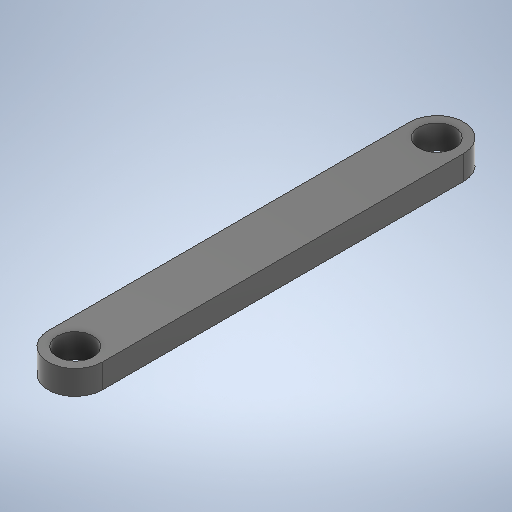
# Autodesk Inventor part: Servo connector
Saved by Autodesk Inventor 2025.2 (Build 292293000, 293)
## iProperties
Created: 2025-01-30
Part Number: Servo connector
Material: Generic
Document SubType Name: Modeling
Designer: caomi
Density: 1 g/cm^3
Appearance: Default
Author: caomi
Autodesk Inventor part; units mm, degrees
ref_plane "YZ Plane" through (0, 0, 0) normal (1, 0, 0) x (0, 1, 0)
ref_plane "XZ Plane" through (0, 0, 0) normal (0, 1, 0) x (-1, 0, 0)
ref_plane "XY Plane" through (0, 0, 0) normal (0, 0, 1) x (1, 0, 0)
sketch "Sketch1" plane through (0, 0, 0) normal (0, 1, 0) x (-1, 0, 0)
  line L0 (0, 15) -> (0, -15) construction
  line L1 (-2.25, 15) -> (-2.25, -15)
  line L2 (2.25, -15) -> (2.25, 15)
  arc A0 (2.25, 15) -> (-2.25, 15) centre (0, 15) ccw
  arc A1 (-2.25, -15) -> (2.25, -15) centre (0, -15) ccw
  circle A2 centre (0, 15) radius 1.5
  circle A3 centre (0, -15) radius 1.5
  point P0 (0, 0)
  dimension "d0" = 4.5
  dimension "d1" = 30
  dimension "d2" = 3
  constraints: 8 end point, 4 centre point, 4 point on circle, 4 tangent, 2 coincident, 1 equal radius, 1 midpoint, 1 parallel, 1 vertical
  measures "d0" distance between parallel lines of L1 L2
  measures "d1" distance of L0.start L0.end
  measures "d2" diameter of A3
extrude "Extrusion1" add sketch "Sketch1" along normal blind 2
body "Solid1"
